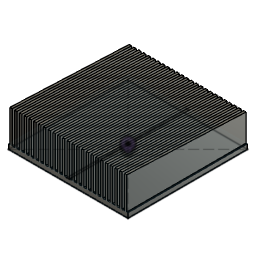
Heat sink v1 (Autodesk Fusion 360 design; units mm, degrees)
Autodesk Fusion 360 part; units mm, degrees
sketch "Sketch1" plane through (0, 0, 0) normal (0, 1, 0) x (1, 0, 0)
  line L0 (31.75, -31.75) -> (-31.75, -31.75)
  line L1 (-31.75, -31.75) -> (-31.75, 31.75)
  line L2 (-31.75, 31.75) -> (31.75, 31.75)
  line L3 (31.75, 31.75) -> (31.75, -31.75)
  line L4 (31.75, -31.75) -> (-31.75, 31.75) construction
  line L5 (-31.75, -31.75) -> (31.75, 31.75) construction
  dimension "d1" = 63.5
  dimension "d2" = 63.5
  constraint horizontal L0
  constraint perpendicular L0 L1
  constraint parallel L0 L2
  constraint parallel L1 L3
  constraint coincident L4 origin
  constraint coincident L5 origin
  measures "d1" distance of L1.end L2.end
  measures "d2" distance of L0.end L1.end
extrude "Extrude1" add sketch "Sketch1" along normal blind 2.54 makes body 1
sketch "Sketch2" plane through (0, 2.54, 0) normal (0, 1, 0) x (-1, 0, 0)
  line L0 (-31.75, -31.75) -> (31.75, -31.75)
  line L1 (31.75, -31.75) -> (31.75, 31.75)
  line L2 (31.75, 31.75) -> (-31.75, 31.75)
  line L3 (-31.75, 31.75) -> (-31.75, -31.75)
  line L4 (0.635, 31.75) -> (-0.635, 31.75)
  line L5 (-0.635, 31.75) -> (-0.635, -31.75)
  line L6 (-0.635, -31.75) -> (0.635, -31.75)
  line L7 (0.635, -31.75) -> (0.635, 31.75)
  line L8 (0.635, 31.75) -> (-0.635, -31.75) construction
  line L9 (-0.635, 31.75) -> (0.635, -31.75) construction
  dimension "d5" = 1.27
  dimension "d6" = 63.5
  constraint horizontal L4
  constraint perpendicular L4 L5
  constraint parallel L4 L6
  constraint parallel L5 L7
  constraint coincident L8 origin
  constraint coincident L9 origin
  measures "d5" distance of L5.end L6.end
  measures "d6" distance of L4.end L5.end
ref_plane "WorkPlane1" through (0.635, 0, 0) normal (1, 0, 0) x (0, 1, 0)
sketch "Fin Shape" plane through (0.635, 0, 0) normal (1, 0, 0) x (0, 0, -1)
  line L0 (31.75, 2.54) -> (-31.75, 2.54)
  line L1 (-31.75, 2.54) -> (-31.75, 16.9038)
  line L2 (-31.75, 16.9038) -> (31.75, 16.9038)
  line L3 (31.75, 16.9038) -> (31.75, 2.54)
  line L4 (31.75, 16.9038) -> (-31.75, 19.6763)
  line L5 (-31.75, 19.6763) -> (-31.75, 16.9038)
  dimension "d14" = 63.5
  dimension "d15" = 14.3638
  dimension "d18" = 2.7725
  constraint horizontal L0
  constraint vertical L1
  constraint horizontal L2
  constraint vertical L3
  constraint perpendicular L2 L5
  measures "d14" distance of L1.end L2.end
  measures "d15" distance of L0.start L2.end
  measures "d18" distance of L1.end L4.end
extrude "Extrude3" add sketch "Fin Shape" against normal blind 1.27 separate body makes body 2
pattern_linear "R-Pattern1" count 25 spacing 2.54 along (1, 0, 0) both ways of bodies 2 makes body 3 at (-29.845, 7.3279, -10.5833) makes body 4 at (-27.305, 7.3279, -10.5833) makes body 5 at (-24.765, 7.3279, -10.5833) makes body 6 at (-22.225, 7.3279, -10.5833) makes body 7 at (-19.685, 7.3279, -10.5833) makes body 8 at (-17.145, 7.3279, -10.5833) makes body 9 at (-14.605, 7.3279, -10.5833) makes body 10 at (-12.065, 7.3279, -10.5833) makes body 11 at (-9.525, 7.3279, -10.5833) makes body 12 at (-6.985, 7.3279, -10.5833) makes body 13 at (-4.445, 7.3279, -10.5833) makes body 14 at (-1.905, 7.3279, -10.5833) makes body 15 at (3.175, 7.3279, -10.5833) makes body 16 at (5.715, 7.3279, -10.5833) makes body 17 at (8.255, 7.3279, -10.5833) makes body 18 at (10.795, 7.3279, -10.5833) makes body 19 at (13.335, 7.3279, -10.5833) makes body 20 at (15.875, 7.3279, -10.5833) makes body 21 at (18.415, 7.3279, -10.5833) makes body 22 at (20.955, 7.3279, -10.5833) makes body 23 at (23.495, 7.3279, -10.5833) makes body 24 at (26.035, 7.3279, -10.5833) makes body 25 at (28.575, 7.3279, -10.5833) makes body 26 at (31.115, 7.3279, -10.5833)
combine "Combine2" operation add target body 1 tool bodies 2 4 25 3 26 19 13 10 11 12 17 20 21 7 9 8 24 23 22 6 5 15 14 16 18
equation "d11 = 1.27 * 2 mm"
